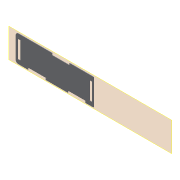
# Autodesk Inventor part: Spacing Layer 4
Saved by Autodesk Inventor 2017 (Build 210142000, 142)
## iProperties
Created: 2016-12-16
Part Number: Spacing Layer 4
Material: Generic
Document SubType Name: Modeling
Designer: Jonis
Density: 1 g/cm^3
Appearance: Default
Author: Jonis
Autodesk Inventor part; units mm, degrees
ref_plane "YZ Plane" through (0, 0, 0) normal (1, 0, 0) x (0, 1, 0)
ref_plane "XZ Plane" through (0, 0, 0) normal (0, 1, 0) x (-1, 0, 0)
ref_plane "XY Plane" through (0, 0, 0) normal (0, 0, 1) x (1, 0, 0)
ref_plane "Work Plane1" through (0, 0, 0) normal (0, 0, 1) x (1, 0, 0)
sketch "Sketch1" plane through (0, 0, 0) normal (0, 0, 1) x (1, 0, 0)
  line L0 (14.7416, 30.2896) -> (14.7416, 47.46) projected
  line L1 (14.7416, 29.7816) -> (14.7416, 30.2896) projected
  line L2 (14.7416, -47.4598) -> (14.7416, 29.7816) projected
  arc A0 (14.7416, 47.46) -> (12.2016, 50) centre (12.2016, 47.46) ccw projected
  line L3 (12.2016, 50) -> (-68.0116, 50) projected
  arc A1 (12.2016, -49.9998) -> (14.7416, -47.4598) centre (12.2016, -47.4598) ccw projected
  line L4 (-6.315, -49.9998) -> (12.2016, -49.9998) projected
  line L5 (-157.7498, -49.9998) -> (-92.5988, -49.9998) projected
  line L6 (-269.9924, -49.9998) -> (-263.9218, -49.9998) projected
  line L7 (-263.9218, -49.9998) -> (-241.9762, -49.9998) projected
  arc A2 (-280, -39.9922) -> (-269.9924, -49.9998) centre (-269.9924, -39.9922) ccw projected
  line L8 (-280, 39.2304) -> (-280, -39.9922) projected
  arc A3 (-269.9924, 50) -> (-280, 39.9924) centre (-269.9924, 39.9924) ccw projected
  line L9 (-280, 39.9924) -> (-280, 39.2304) projected
  line L10 (-263.4646, 50) -> (-269.9924, 50) projected
  line L11 (-152.238, 50) -> (-263.4646, 50) projected
  line L12 (-152.238, 50) -> (-68.0116, 50)
  line L13 (-92.5988, -49.9998) -> (-6.315, -49.9998)
  line L14 (-157.7498, -49.9998) -> (-241.9762, -49.9998)
  point P0 (0, 0)
  constraints: 6 end point, 1 collinear, 1 horizontal, 1 parallel
extrude "Extrusion1" add sketch "Sketch1" along normal blind 1.6
sketch "Sketch2" plane through (0, 0, 1.6) normal (0, 0, 1) x (1, 0, 0)
  circle A0 centre (0.1366, 35.649) radius 1.75 projected
  circle A1 centre (-13.046, 44.1326) radius 1.75 projected
  circle A2 centre (0.1366, -38.011) radius 1.75 projected
  circle A3 centre (-13.046, -44.107) radius 1.75 projected
  circle A4 centre (-73.2948, 44.1072) radius 1.75 projected
  circle A5 centre (-86.706, -44.107) radius 1.75 projected
  circle A6 centre (-146.9548, 44.1072) radius 1.75 projected
  circle A7 centre (-163.033, -44.107) radius 1.75 projected
  circle A8 centre (-250.0026, -44.107) radius 1.75 projected
  circle A9 centre (-271.3132, -38.011) radius 1.75 projected
  circle A10 centre (-236.693, -44.107) radius 1.75 projected
  circle A11 centre (-271.3132, 35.649) radius 1.75 projected
  circle A12 centre (-250.0026, 44.1326) radius 1.75 projected
  point P0 (0, 0)
  constraints: 13 coincident
hole "Hole1" at (0.1366, 35.649, 1.6) at (-13.046, 44.1326, 1.6) at (0.1366, -38.011, 1.6) at (-13.046, -44.107, 1.6) at (-86.706, -44.107, 1.6) at (-146.9548, 44.1072, 1.6) at (-163.033, -44.107, 1.6) at (-236.693, -44.107, 1.6) at (-250.0026, -44.107, 1.6) at (-271.3132, -38.011, 1.6) at (-271.3132, 35.649, 1.6) at (-250.0026, 44.1326, 1.6) at (-73.2948, 44.1072, 1.6) direction (0, 0, -1) diameter 1.6 depth 5 tip angle 118
sketch "Sketch3" plane through (0, 0, 1.6) normal (0, 0, 1) x (1, 0, 0)
  line L0 (8.922, 31.9915) -> (8.922, -34.5585) projected
  line L1 (-0.978, 31.9915) -> (8.922, 31.9915) projected
  line L2 (-0.978, 31.9915) -> (-0.978, -34.5585) projected
  line L3 (8.922, -34.5585) -> (-0.978, -34.5585) projected
  line L4 (-76.7473, 52.8925) -> (-76.7473, 42.9925) projected
  line L5 (-143.2973, 52.8925) -> (-76.7473, 52.8925) projected
  line L6 (-143.2973, 42.9925) -> (-76.7473, 42.9925) projected
  line L7 (-143.2973, 42.9925) -> (-143.2973, 52.8925) projected
  line L8 (-16.7036, -42.9923) -> (-16.7036, -52.8923) projected
  line L9 (-16.7036, -52.8923) -> (-83.2536, -52.8923) projected
  line L10 (-16.7036, -42.9923) -> (-83.2536, -42.9923) projected
  line L11 (-83.2536, -52.8923) -> (-83.2536, -42.9923) projected
  line L12 (-166.6905, -42.9923) -> (-233.2405, -42.9923) projected
  line L13 (-166.6905, -52.8923) -> (-233.2405, -52.8923) projected
  line L14 (-233.2405, -52.8923) -> (-233.2405, -42.9923) projected
  line L15 (-166.6905, -42.9923) -> (-166.6905, -52.8923) projected
  line L16 (-262.5279, 31.9915) -> (-262.5279, -34.5585) projected
  line L17 (-272.4279, 31.9915) -> (-262.5279, 31.9915) projected
  line L18 (-272.4279, 31.9915) -> (-272.4279, -34.5585) projected
  line L19 (-262.5279, -34.5585) -> (-272.4279, -34.5585) projected
  point P0 (0, 0)
extrude "Extrusion2" cut sketch "Sketch3" against normal blind 1.6
body "Solid1"
